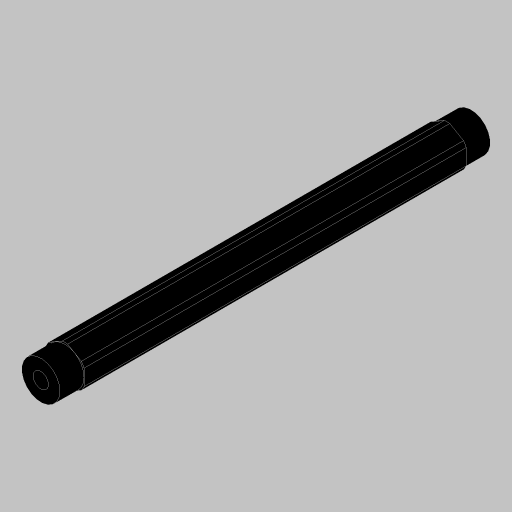
# Autodesk Inventor part: CL4-019
Saved by Autodesk Inventor 2023.5 (Build 275446000, 446)
## iProperties
RuleStatus: InUse
Created: 2025-02-05
Part Number: CL4-019
Material: Aluminum 6061
Document SubType Name: Modeling
Designer: brand
Mass: 8.50758 g
Surface Area: 25.7449 cm^2
Volume: 3.15096 cm^3
Density: 2.7 g/cm^3
Appearance: Anodized - Black
AfterDocNew0: SHOW
AfterDocOpen0: SHOW
AfterDocOpen1: size
AfterDocOpen2: thunder
BeforeDocSave0: size
BeforeDocSave1: thunder
AfterFeatureSuppressionChange0: thunder
AfterFeatureSuppressionChange1: size
PartBodyChanged0: thunder
PartBodyChanged1: size
AfterMaterialChange0: thunder
AfterMaterialChange1: size
Author: brand
Autodesk Inventor part; units mm, degrees
ref_plane "YZ Plane" through (0, 0, 0) normal (1, 0, 0) x (0, 1, 0)
ref_plane "XZ Plane" through (0, 0, 0) normal (0, 1, 0) x (-1, 0, 0)
ref_plane "XY Plane" through (0, 0, 0) normal (0, 0, 1) x (1, 0, 0)
sketch "Sketch1" plane through (0, 0, 0) normal (0, 0, 1) x (1, 0, 0)
  line L0 (-6.35, -3.666174) -> (-6.35, 3.666174)
  line L1 (-6.35, 3.666174) -> (0, 7.332348)
  line L2 (0, 7.332348) -> (6.35, 3.666174)
  line L3 (6.35, 3.666174) -> (6.35, -3.666174)
  line L4 (6.35, -3.666174) -> (0, -7.332348)
  line L5 (0, -7.332348) -> (-6.35, -3.666174)
  point P0 (0, 0)
  point P1 (0, 0)
  dimension "Size" = 12.7
  constraints: 12 end point, 1 coincident, 1 vertical alignment, 13 other
  measures "Size" distance between parallel lines of L3 L0
extrude "Extrusion1" add sketch "Sketch1" along normal mid plane 142.875
sketch "Sketch3" plane through (0, 0, 71.4375) normal (0, 0, 1) x (1, 0, 0)
  line L0 (-6.35, 3.666174) -> (0, 7.332348) construction
  line L1 (0, 7.332348) -> (6.35, 3.666174) construction
  line L2 (6.35, 3.666174) -> (6.35, -3.666174) construction
  line L3 (6.35, -3.666174) -> (0, -7.332348) construction
  line L4 (0, -7.332348) -> (-6.35, -3.666174) construction
  line L5 (-6.35, -3.666174) -> (-6.35, 3.666174) construction
  point P0 (0, 0)
hole "Hole1" at (0, 0, 71.4375) direction (0, 0, -1) diameter 5.1054 end through all
sketch "Sketch4" plane through (0, 0, 71.4375) normal (0, 0, 1) x (1, 0, 0)
  circle A0 centre (0, 0) radius 2.5527 construction
  line L0 (-6.35, 3.666174) -> (0, 7.332348) construction
  line L1 (0, 7.332348) -> (6.35, 3.666174) construction
  line L2 (6.35, 3.666174) -> (6.35, -3.666174) construction
  line L3 (6.35, -3.666174) -> (0, -7.332348) construction
  line L4 (0, -7.332348) -> (-6.35, -3.666174) construction
  line L5 (-6.35, -3.666174) -> (-6.35, 3.666174) construction
  circle A1 centre (0, 0) radius 6.87705
  circle A2 centre (0, 0) radius 8.89
  dimension "thunder" = 13.7541
  dimension "d16" = 17.78
  constraints: 2 centre point, 2 coincident
  measures "thunder" diameter of A1
  measures "d16" diameter of A2
extrude "Extrusion3" cut sketch "Sketch4" against normal through all
sketch "Sketch5" plane through (0, 0, 71.4375) normal (0, 0, 1) x (1, 0, 0)
  arc A0 (5.461589, -4.179099) -> (6.35, -2.640325) centre (0, 0) ccw
  line L0 (5.461589, -4.179099) -> (0.888411, -6.819424)
  arc A1 (-0.888411, -6.819424) -> (0.888411, -6.819424) centre (0, 0) ccw
  line L1 (-0.888411, -6.819424) -> (-5.461589, -4.179099)
  arc A2 (-6.35, -2.640325) -> (-5.461589, -4.179099) centre (0, 0) ccw
  line L2 (-6.35, -2.640325) -> (-6.35, 2.640325)
  arc A3 (-5.461589, 4.179099) -> (-6.35, 2.640325) centre (0, 0) ccw
  line L3 (-5.461589, 4.179099) -> (-0.888411, 6.819424)
  arc A4 (0.888411, 6.819424) -> (-0.888411, 6.819424) centre (0, 0) ccw
  line L4 (0.888411, 6.819424) -> (5.461589, 4.179099)
  arc A5 (6.35, 2.640325) -> (5.461589, 4.179099) centre (0, 0) ccw
  line L5 (6.35, 2.640325) -> (6.35, -2.640325)
  circle A6 centre (0, 0) radius 2.5527
  circle A7 centre (0, 0) radius 6.35
  point P0 (-3.175, 5.499261)
  point P1 (3.175, 5.499261)
  point P2 (6.35, 0)
  point P3 (-6.35, 0)
  point P4 (-3.175, -5.499261)
  point P5 (3.175, -5.499261)
  dimension "d19" = 12.7
  constraints: 1 centre point, 1 coincident
  measures "d19" diameter of A7
extrude "Extrusion4" cut sketch "Sketch5" against normal blind 8.001 contours L0 A7 L5 A0 | L0 A1 L1 A7 | A7 L4 A5 L5 | L1 A2 L2 A7 | A7 L3 A4 L4 | L2 A3 L3 A7
mirror "Mirror2" about plane through (0, 0, 0) normal (0, 0, 1) of "Extrusion4"
equation "\"bearing\" = 25.4"
body "Solid1"
